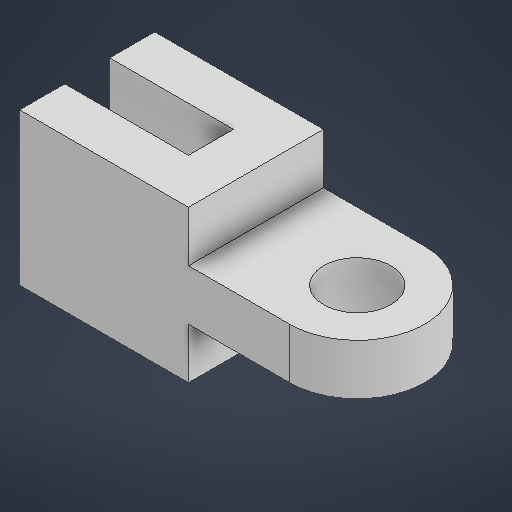
# Autodesk Inventor part: Part7
Saved by Autodesk Inventor 2026 (Build 300175050, 175E)
## iProperties
Created: 2026-03-19
Part Number: Part7
Material: Generic
Document SubType Name: Modeling
Designer: Administrator
Density: 1 g/cm^3
Appearance: Default
Author: Administrator
Autodesk Inventor part; units mm, degrees
ref_plane "YZ Plane" through (0, 0, 0) normal (1, 0, 0) x (0, 1, 0)
ref_plane "XZ Plane" through (0, 0, 0) normal (0, 1, 0) x (-1, 0, 0)
ref_plane "XY Plane" through (0, 0, 0) normal (0, 0, 1) x (1, 0, 0)
sketch "Sketch1" plane through (0, 0, 0) normal (0, 0, 1) x (1, 0, 0)
  line L0 (0, 0) -> (60, 0)
  line L1 (60, 0) -> (60, 27)
  line L2 (60, 27) -> (0, 27)
  line L3 (0, 27) -> (0, 0)
  dimension "d0" = 27
  dimension "d1" = 60
  constraints: 8 end point, 3 perpendicular, 1 horizontal
  measures "d0" distance of L2.end L0.start
  measures "d1" distance of L1.end L2.end
extrude "Extrusion1" add sketch "Sketch1" along normal mid plane 24
sketch "Sketch2" plane through (0, 27, 12) normal (0, 1, 0) x (1, 0, 0)
  line L0 (30, 26.8485) -> (66.8561, 26.8485)
  line L1 (66.8561, 26.8485) -> (66.8561, -1.1061)
  line L2 (66.8561, -1.1061) -> (30, -1.1061)
  line L3 (30, -1.1061) -> (30, 26.8485)
  line L4 (0, 24) -> (0, 0) projected
  point P0 (0, 12)
  dimension "d4" = 30
  constraints: 8 end point, 2 parallel, 1 horizontal, 1 perpendicular
  measures "d4" distance between parallel lines of L4 L3
extrude "Extrusion2" cut sketch "Sketch2" against normal blind 9
sketch "Sketch3" plane through (0, 0, 12) normal (0, -1, 0) x (1, 0, 0)
  line L0 (64.8246, 8.5283) -> (30, 8.5283)
  line L1 (30, 8.5283) -> (30, -38.3826)
  line L2 (30, -38.3826) -> (64.8246, -38.3826)
  line L3 (64.8246, -38.3826) -> (64.8246, 8.5283)
  line L4 (0, -24) -> (0, 0) projected
  point P0 (0, -12)
  dimension "d7" = 30
  constraints: 8 end point, 2 parallel, 1 horizontal, 1 perpendicular
  measures "d7" distance between parallel lines of L4 L1
extrude "Extrusion3" cut sketch "Sketch3" against normal blind 9
sketch "Sketch4" plane through (0, 18, 12) normal (0, 1, 0) x (1, 0, 0)
  circle A0 centre (48, 12) radius 6
  line L0 (30, 0) -> (30, 24) projected
  line L1 (30, 24) -> (60, 24) projected
  point P0 (0, 12)
  dimension "d10" = 12
  dimension "d11" = 18
  dimension "d12" = 12
  constraints: 1 centre point
  measures "d10" diameter of A0
  measures "d11" distance from line of L0 A0.centre
  measures "d12" distance from line of L1 A0.centre
extrude "Extrusion4" cut sketch "Sketch4" against normal blind 9
fillet "Fillet1" radius 12 1 edges at (60, 13.5, 12)
fillet "Fillet2" radius 12 1 edges at (60, 13.5, -12)
sketch "Sketch5" plane through (0, 27, 12) normal (0, 1, 0) x (1, 0, 0)
  line L0 (0, 16) -> (22, 16)
  line L1 (22, 16) -> (22, 8)
  line L2 (22, 8) -> (0, 8)
  line L3 (0, 8) -> (0, 16)
  line L4 (0, 24) -> (30, 24) projected
  line L5 (30, 0) -> (0, 0) projected
  line L6 (30, 0) -> (30, 24) projected
  point P0 (0, 12)
  dimension "d17" = 8
  dimension "d18" = 8
  dimension "d19" = 8
  dimension "d20" = 22
  constraints: 8 end point, 2 parallel, 1 horizontal, 1 perpendicular
  measures "d17" distance between parallel lines of L4 L0
  measures "d18" distance between parallel lines of L5 L2
  measures "d19" distance between parallel lines of L6 L1
  measures "d20" distance between parallel lines of L1 L3
extrude "Extrusion5" cut sketch "Sketch5" against normal blind 27
body "Solid1"
